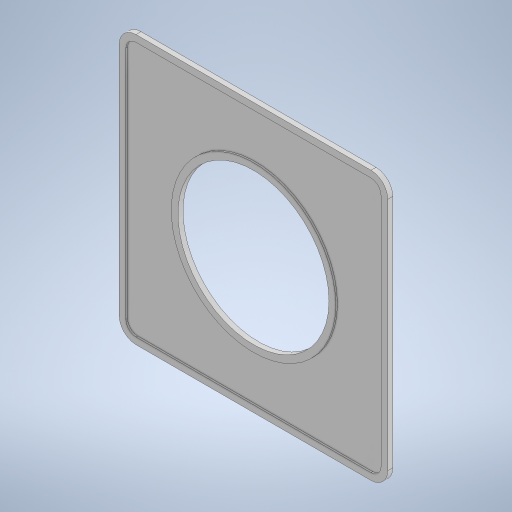
# Autodesk Inventor part: Parte2
Saved by Autodesk Inventor 2024 (Build 280153000, 153)
## iProperties
Created: 2023-12-17
Part Number: Parte2
Material: Generico
Document SubType Name: Modeling
Designer: cecca
Density: 1 g/cm^3
Appearance: Default
Author: cecca
Autodesk Inventor part; units mm, degrees
ref_plane "YZ Plane" through (0, 0, 0) normal (1, 0, 0) x (0, 1, 0)
ref_plane "XZ Plane" through (0, 0, 0) normal (0, 1, 0) x (-1, 0, 0)
ref_plane "XY Plane" through (0, 0, 0) normal (0, 0, 1) x (1, 0, 0)
sketch "Schizzo1" plane through (0, 0, 0) normal (0, 0, 1) x (1, 0, 0)
  line L0 (40, -40) -> (-40, -40)
  line L1 (-40, -40) -> (-40, 40)
  line L2 (-40, 40) -> (40, 40)
  line L3 (40, 40) -> (40, -40)
  line L4 (40, -40) -> (-40, 40) construction
  line L5 (-40, -40) -> (40, 40) construction
  circle A0 centre (0, 0) radius 22.5
  dimension "d0" = 80
  dimension "d1" = 80
  dimension "d2" = 45
  constraints: 12 end point, 2 midpoint, 2 parallel, 1 centre point, 1 coincident, 1 horizontal, 1 perpendicular
  measures "d0" distance of L1.end L2.end
  measures "d1" distance of L0.end L1.end
  measures "d2" diameter of A0
extrude "Estrusione1" add sketch "Schizzo1" along normal mid plane 1.5
fillet "Raccordo1" radius 5 4 edges at (40, 40, 0) (40, -40, 0) (-40, -40, 0) (-40, 40, 0)
sketch "Schizzo2" plane through (0, 0, 0.75) normal (0, 0, 1) x (1, 0, 0)
  line L0 (35, -40) -> (-35, -40) projected
  line L1 (0, -40) -> (0, -38)
  line L2 (0, -38) -> (35, -38)
  line L3 (0, -38) -> (-35, -38)
  line L4 (-40, -35) -> (-40, 35) projected
  line L5 (-40, 0) -> (-38, 0)
  line L6 (-38, 0) -> (-38, -35)
  arc A0 (-38, -35) -> (-35, -38) centre (-35, -35) ccw
  line L7 (40, 35) -> (40, -35) projected
  line L8 (0, 38) -> (35, 38)
  line L9 (0, 38) -> (-35, 38)
  line L10 (-38, 0) -> (-38, 35)
  arc A1 (-35, 38) -> (-38, 35) centre (-35, 35) ccw
  line L11 (35, 40) -> (-35, 40) projected
  line L12 (38, 0) -> (38, 35)
  arc A2 (38, 35) -> (35, 38) centre (35, 35) ccw
  line L13 (38, 0) -> (38, -35)
  arc A3 (35, -38) -> (38, -35) centre (35, -35) ccw
  circle A4 centre (0, 0) radius 24.5
  dimension "d6" = 2
  dimension "d8" = 35
  dimension "d9" = 35
  dimension "d10" = 2
  dimension "d11" = 35
  constraints: 20 end point, 8 point on circle, 5 centre point, 3 horizontal, 2 midpoint, 1 coincident, 1 perpendicular, 1 vertical
  measures "d6" distance of L1.start L1.end
  measures "d8" distance of L1.end L2.end
  measures "d9" distance of L1.end L3.end
  measures "d10" distance of L5.start L5.end
  measures "d11" distance of L5.end L6.end
extrude "Estrusione2" cut sketch "Schizzo2" against normal blind 0.5
